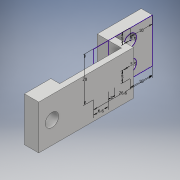
# Autodesk Inventor part: Laser_Holder
Saved by Autodesk Inventor 2017 (Build 210142000, 142)
## iProperties
Created: 2017-03-24
Part Number: Laser_Holder
Material: Generic
Document SubType Name: Modeling
Designer: willt
Density: 1 g/cm^3
Appearance: Default
Author: willt
Autodesk Inventor part; units mm, degrees
ref_plane "YZ Plane" through (0, 0, 0) normal (1, 0, 0) x (0, 1, 0)
ref_plane "XZ Plane" through (0, 0, 0) normal (0, 1, 0) x (-1, 0, 0)
ref_plane "XY Plane" through (0, 0, 0) normal (0, 0, 1) x (1, 0, 0)
sketch "Sketch1" plane through (0, 0, 0) normal (1, 0, 0) x (0, 1, 0)
  line L0 (0, 0) -> (-26.6, 0)
  line L1 (-26.6, 0) -> (-26.6, -20)
  line L2 (-26.6, -20) -> (0, -20)
  line L3 (0, -20) -> (0, 0)
  line L4 (0, 0) -> (-10, 0) construction
  line L5 (-10, 0) -> (-10, -5) construction
  circle A0 centre (-10, -5) radius 2.75
  line L6 (0, -20) -> (-10, -20) construction
  line L7 (-10, -20) -> (-10, -15) construction
  circle A1 centre (-10, -15) radius 2.75
  line L8 (-26.6, 0) -> (-20, 0)
  line L9 (-20, 0) -> (-20, -20)
  line L10 (-20, -20) -> (-26.6, -20)
  line L11 (-26.6, -20) -> (-26.6, 0)
  line L12 (-20, 0) -> (-17, 0)
  line L13 (-17, 0) -> (-17, -20)
  line L14 (-17, -20) -> (-20, -20)
  line L15 (-20, -20) -> (-20, 0)
  dimension "d0" = 26.6
  dimension "d1" = 20
  dimension "d2" = 10
  dimension "d3" = 5
  dimension "d4" = 5.5
  dimension "d5" = 10
  dimension "d6" = 5
  dimension "d7" = 5.5
  dimension "d8" = 6.6
  dimension "d9" = 3
  constraints: 32 end point, 6 parallel, 5 perpendicular, 4 point on line, 3 horizontal, 2 centre point, 2 coincident
  measures "d0" distance of L2.end L1.end
  measures "d1" distance of L1.end L0.end
  measures "d2" distance of L0.start L4.end
  measures "d3" distance of L4.end L5.end
  measures "d4" diameter of A0
  measures "d5" distance of L2.end L6.end
  measures "d6" distance of L6.end L7.end
  measures "d7" diameter of A1
  measures "d8" distance of L9.end L10.end
  measures "d9" distance of L13.end L14.end
extrude "Extrusion1" add sketch "Sketch1" along normal blind 8.5 contours L13 L2 L9 L0
extrude "Extrusion2" add sketch "Sketch1" against normal blind 5 contours L3 L2 L13 L0
extrude "Extrusion3" add sketch "Sketch1" against normal blind 5 contours L13 L2 L9 L0
sketch "Sketch2" plane through (8.5, -20, -20) normal (0, -1, 0) x (1, 0, 0)
  line L0 (0, 20) -> (0, 0) projected
  line L1 (-8.5, 0) -> (0, 0) projected
  line L2 (0, 20) -> (-2.5, 20)
  line L3 (-2.5, 20) -> (-2.5, 0)
  line L4 (-2.5, 0) -> (0, 0)
  line L5 (0, 0) -> (0, 20)
  point P0 (-8.5, 20)
  dimension "d16" = 2.5
  constraints: 8 end point, 2 parallel, 1 horizontal, 1 perpendicular, 1 point on line
  measures "d16" distance of L4.end L3.end
extrude "Extrusion4" add sketch "Sketch2" along normal blind 40
sketch "Sketch3" plane through (8.5, 0, 0) normal (1, 0, 0) x (0, 0, -1)
  line L0 (20, -60) -> (0, -60) projected
  circle A0 centre (10, -54) radius 3
  point P0 (0, 0)
  dimension "d20" = 6
  constraints: 1 centre point
  measures "d20" diameter of A0
extrude "Extrusion5" cut sketch "Sketch3" against normal blind 7.5
sketch "Sketch4" plane through (6, -20, -20) normal (-1, 0, 0) x (0, 0, 1)
  line L0 (20, 3) -> (20, -40) projected
  line L1 (0, 3) -> (0, -40) projected
  line L2 (20, -40) -> (0, -40)
  line L3 (0, -40) -> (0, -28)
  line L4 (0, -28) -> (20, -28)
  line L5 (20, -28) -> (20, -40)
  point P0 (20, 20)
  dimension "d23" = 12
  constraints: 8 end point, 2 parallel, 1 horizontal, 1 perpendicular, 1 point on line
  measures "d23" distance of L2.end L3.end
extrude "Extrusion6" add sketch "Sketch4" along normal blind 4
sketch "Sketch5" plane through (6, -54, -10) normal (1, 0, 0) x (0, 0, -1)
  circle A0 centre (0, 0) radius 3
  point P0 (-10, 54)
  constraints: 1 centre point
extrude "Extrusion7" cut sketch "Sketch5" against normal blind 4
body "Solid1"
